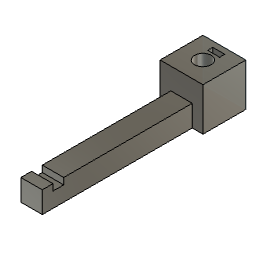
Piece for weight holding (Autodesk Fusion 360 design; units mm, degrees)
Autodesk Fusion 360 part; units mm, degrees
sketch "Esquisse1" plane through (0, 0, 0) normal (0, 0, 1) x (1, 0, 0)
sketch "Esquisse2" plane through (0, 0, 0) normal (0, 0, 1) x (1, 0, 0)
  circle A0 centre (0, 0) radius 3.865
  line L0 (10, -10) -> (-10, -10)
  line L1 (-10, -10) -> (-10, 10)
  line L2 (-10, 10) -> (10, 10)
  line L3 (10, 10) -> (10, -10)
  dimension "d2" = 7.73
  constraint coincident A0.centre origin
  constraint horizontal L0
  constraint vertical L1
  constraint horizontal L2
  constraint vertical L3
  measures "d2" diameter of A0
extrude "Extrusion1" add sketch "Esquisse2" along normal blind 20
sketch "Esquisse3" plane through (0, 10, 0) normal (0, 1, 0) x (-1, 0, 0)
  line L0 (-10, 0) -> (10, 0)
  line L1 (10, 0) -> (10, 20)
  line L2 (10, 20) -> (-10, 20)
  line L3 (-10, 20) -> (-10, 0)
sketch "Esquisse4" plane through (0, 0, 20) normal (0, 0, 1) x (-1, 0, 0)
  circle A0 centre (0, 0) radius 3.865
  line L0 (-10, -10) -> (10, -10)
  line L1 (10, -10) -> (10, 10)
  line L2 (10, 10) -> (-10, 10)
  line L3 (-10, 10) -> (-10, -10)
  line L4 (0, -7.4) -> (2.8, -7.4)
  line L5 (2.8, -7.4) -> (2.8, -5)
  line L6 (2.8, -5) -> (-2.8, -5)
  line L7 (-2.8, -5) -> (-2.8, -7.4)
  line L8 (-2.8, -7.4) -> (0, -7.4)
  dimension "d12" = 2.8
  dimension "d13" = 5.6
  constraint perpendicular L4 L5
  constraint perpendicular L6 L7
  measures "d12" distance of L4.start L4.end
  measures "d13" distance of L5.end L6.end
ref_plane "Plan de construction1" through (0, 0, 20) normal (0, 1, 0) x (-1, 0, 0)
sketch "Esquisse5" plane through (0, 0, 20) normal (0, 1, 0) x (-1, 0, 0)
  line L0 (0, 0) -> (0, -20)
  line L1 (-10, -10) -> (10, -10)
  line L2 (0, -6.8) -> (-2.7713, -8.4)
  line L3 (-2.7713, -8.4) -> (-2.7713, -11.6)
  line L4 (-2.7713, -11.6) -> (0, -13.2)
  line L5 (0, -13.2) -> (2.7713, -11.6)
  line L6 (2.7713, -11.6) -> (2.7713, -8.4)
  line L7 (2.7713, -8.4) -> (0, -6.8)
  point P0 (0, -10)
  dimension "d6" = 3.2
  constraint coincident L0.start origin
  constraint vertical L0
  constraint horizontal L1
  constraint midpoint L1 P0
  measures "d6" distance of L2.start P0
extrude "Extrusion2" cut sketch "Esquisse5" along normal blind 2.4 from surface at 5
extrude "Extrusion3" cut sketch "Esquisse4" against normal blind 9 contours L4 L5 L6 L7 L8
sketch "Esquisse6" plane through (0, 10, 0) normal (0, 1, 0) x (-1, 0, 0)
  circle A0 centre (0, 10) radius 1.625
  dimension "d16" = 3.25
  measures "d16" diameter of A0
extrude "Extrusion4" cut sketch "Esquisse6" against normal blind 10
sketch "Esquisse7" plane through (0, -10, 0) normal (0, -1, 0) x (1, 0, 0)
  line L0 (-10, 0) -> (10, 0)
  line L1 (10, 0) -> (10, 20)
  line L2 (10, 20) -> (-10, 20)
  line L3 (-10, 20) -> (-10, 0)
  line L4 (5, 15) -> (-5, 15)
  line L5 (-5, 15) -> (-5, 5)
  line L6 (-5, 5) -> (5, 5)
  line L7 (5, 5) -> (5, 15)
  line L8 (5, 15) -> (-5, 5) construction
  line L9 (-5, 15) -> (5, 5) construction
  point P0 (0, 10)
  dimension "d19" = 10
  dimension "d20" = 10
  constraint horizontal L4
  constraint perpendicular L4 L5
  constraint parallel L4 L6
  constraint parallel L5 L7
  constraint coincident L8 P0
  constraint coincident L9 P0
  measures "d19" distance of L5.end L6.end
  measures "d20" distance of L4.end L5.end
extrude "Extrusion5" add sketch "Esquisse7" along normal blind 70 contours L4 L5 L6 L7
sketch "Esquisse8" plane through (0, 0, 15) normal (0, 0, 1) x (-1, 0, 0)
  line L0 (-5, 10) -> (5, 10)
  line L1 (5, 10) -> (5, 80)
  line L2 (5, 80) -> (-5, 80)
  line L3 (-5, 80) -> (-5, 10)
  line L4 (5, 80) -> (-5, 80)
  line L5 (-5, 80) -> (-5, 75)
  line L6 (-5, 75) -> (5, 75)
  line L7 (5, 75) -> (5, 80)
  line L8 (-5, 75) -> (5, 75)
  line L9 (5, 75) -> (5, 70)
  line L10 (5, 70) -> (-5, 70)
  line L11 (-5, 70) -> (-5, 75)
  constraint horizontal L4
  constraint vertical L5
  constraint horizontal L6
  constraint vertical L7
  constraint coincident L3 L5.end
  constraint coincident L1.end L2.start
  constraint horizontal L8
  constraint vertical L9
  constraint horizontal L10
  constraint vertical L11
  constraint coincident L1 L9.end
extrude "Extrusion6" cut sketch "Esquisse8" against normal blind 3 contours L1 L3 L6 L8 L9 L10 L11
extrude "Extrusion7" add 1 faces at (-1.6667, -33.3333, 5) along direction (0, 0, -1) blind 5
extrude "Extrusion8" cut 2 faces at (1.6667, -50, 15) (1.6667, -76.6667, 15) along direction (0, 0, -1) blind 5
extrude "Extrusion9" cut 1 faces at (-1.6667, -71.6667, 12) along direction (0, 0, -1) blind 5
